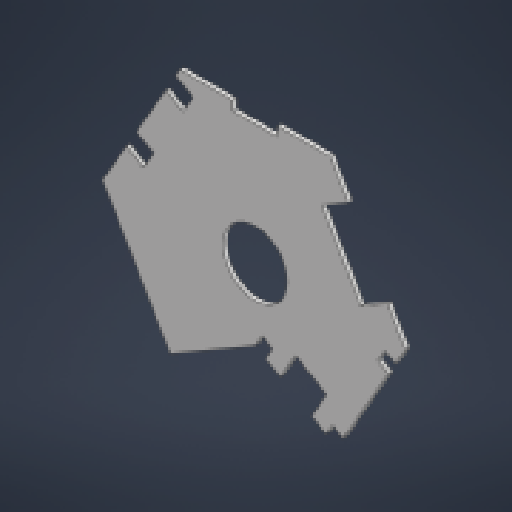
# Autodesk Inventor part: LilypadPCB
Saved by Autodesk Inventor 2023 (Build 270158000, 158)
## iProperties
Created: 2022-07-15
Part Number: LilypadPCB
Material: Generic
Document SubType Name: Modeling
Designer: jevan
Density: 1 g/cm^3
Appearance: Default
Author: jevan
Autodesk Inventor part; units mm, degrees
ref_plane "YZ Plane" through (0, 0, 0) normal (1, 0, 0) x (0, 1, 0)
ref_plane "XZ Plane" through (0, 0, 0) normal (0, 1, 0) x (-1, 0, 0)
ref_plane "XY Plane" through (0, 0, 0) normal (0, 0, 1) x (1, 0, 0)
sketch "Sketch1" plane through (0, 0, 0) normal (0, 0, 1) x (1, 0, 0)
  line L0 (37.2391, 0) -> (18.6195, -32.25)
  line L1 (18.6195, -32.25) -> (-18.6195, -32.25)
  line L2 (-18.6195, -32.25) -> (-37.2391, 0)
  line L3 (-37.2391, 0) -> (-18.6195, 32.25)
  line L4 (-18.6195, 32.25) -> (18.6195, 32.25)
  line L5 (18.6195, 32.25) -> (37.2391, 0)
  line L6 (18.6195, -32.25) -> (20.2545, -29.4181)
  line L7 (20.2545, -29.4181) -> (0, -17.7241)
  line L8 (0, -17.7241) -> (-20.2545, -29.4181)
  line L9 (-20.2545, -29.4181) -> (-21.1206, -29.9181)
  line L10 (-21.1206, -29.9181) -> (-37.8164, -1)
  line L11 (-37.8164, -1) -> (-37.2391, 0)
  circle A0 centre (0, 0) radius 8
  line L12 (-37.8164, -1) -> (-31.9414, 9.1758)
  line L13 (-31.9414, 9.1758) -> (-27.6806, 6.7158)
  line L14 (-27.6806, 6.7158) -> (-25.1806, 11.0459)
  line L15 (-25.1806, 11.0459) -> (-29.4414, 13.5059)
  line L16 (-29.4414, 13.5059) -> (-22.1914, 26.0633)
  line L17 (-22.1914, 26.0633) -> (-17.9133, 23.5933)
  line L18 (-17.9133, 23.5933) -> (-15.4133, 27.9234)
  line L19 (-15.4133, 27.9234) -> (-19.6914, 30.3934)
  line L20 (0, 32.25) -> (5.55, 32.25)
  line L21 (0, 32.25) -> (-5.55, 32.25)
  line L22 (-5.55, 32.25) -> (-5.55, 29.94)
  line L23 (-5.55, 29.94) -> (5.55, 29.94)
  line L24 (5.55, 29.94) -> (5.55, 32.25)
  line L25 (27.9293, 16.125) -> (32.7793, 7.7246)
  line L26 (27.9293, 16.125) -> (23.0793, 24.5254)
  line L27 (23.0793, 24.5254) -> (16.4975, 20.7254)
  line L28 (16.4975, 20.7254) -> (26.1975, 3.9246)
  line L29 (26.1975, 3.9246) -> (32.7793, 7.7246)
  line L30 (37.2391, 0) -> (34.7641, -4.2868)
  line L31 (34.7641, -4.2868) -> (32.1227, -2.7618)
  line L32 (32.1227, -2.7618) -> (30.4227, -5.7063)
  line L33 (30.4227, -5.7063) -> (33.0641, -7.2313)
  line L34 (33.0641, -7.2313) -> (21.8141, -26.7169)
  line L35 (21.8141, -26.7169) -> (19.1641, -25.1869)
  line L36 (19.1641, -25.1869) -> (17.6045, -27.8881)
  line L37 (10.1273, -23.5711) -> (13.9984, -25.8061)
  line L38 (10.1273, -23.5711) -> (6.2561, -21.3361)
  line L39 (6.2561, -21.3361) -> (9.9861, -14.8756)
  line L40 (9.9861, -14.8756) -> (17.7284, -19.3456)
  line L41 (17.7284, -19.3456) -> (13.9984, -25.8061)
  line L42 (6.2561, -21.3361) -> (2.6015, -19.2261)
  line L43 (2.6015, -19.2261) -> (4.3015, -16.2816)
  line L44 (4.3015, -16.2816) -> (1.7, -14.7796)
  line L45 (1.7, -14.7796) -> (0, -17.7241)
  dimension "d0" = 64.5
  dimension "d1" = 3.27
  dimension "d2" = 1
  dimension "d3" = 16
  dimension "d4" = 11.75
  dimension "d5" = 4.92
  dimension "d6" = 5
  dimension "d7" = 14.5
  dimension "d8" = 4.94
  dimension "d9" = 5
  dimension "d10" = 5.55
  dimension "d11" = 5.55
  dimension "d12" = 2.31
  dimension "d13" = 9.7
  dimension "d14" = 9.7
  dimension "d15" = 7.6
  dimension "d16" = 4.95
  dimension "d17" = 3.05
  dimension "d18" = 3.4
  dimension "d19" = 22.5
  dimension "d21" = 3.06
  dimension "d22" = 4.47
  dimension "d23" = 4.47
  dimension "d24" = 7.46
  dimension "d25" = 4.22
  dimension "d26" = 3.4
  constraints: 92 end point, 25 perpendicular, 19 point on line, 3 midpoint, 2 coincident, 2 parallel, 1 centre point, 1 equal length, 1 horizontal, 13 other
  measures "d0" distance between parallel lines of L3 L0
  measures "d1" distance of L0.end L6.end
  measures "d2" distance of L8.end L9.end
  measures "d3" diameter of A0
  measures "d4" distance of L10.end L12.end
  measures "d5" distance of L12.end L13.end
  measures "d6" distance of L13.end L14.end
  measures "d7" distance of L15.end L16.end
  measures "d8" distance of L16.end L17.end
  measures "d9" distance of L17.end L18.end
  measures "d10" distance of L20.start L20.end
  measures "d11" distance of L20.start L21.end
  measures "d12" distance of L21.end L22.end
  measures "d13" distance of L25.start L25.end
  measures "d14" distance of L25.start L26.end
  measures "d15" distance of L26.end L27.end
  measures "d16" distance of L0.start L30.end
  measures "d17" distance of L30.end L31.end
  measures "d18" distance of L31.end L32.end
  measures "d19" distance of L33.end L34.end
  measures "d21" distance of L34.end L35.end
  measures "d22" distance of L37.start L37.end
  measures "d23" distance of L37.start L38.end
  measures "d24" distance of L38.end L39.end
  measures "d25" distance of L38.end L42.end
  measures "d26" distance of L42.end L43.end
extrude "Extrusion1" add sketch "Sketch1" along normal blind 1 contours L0 L31 L32 L33 L35 L36 L7 L41 L40 L39 L43 L44 L45 L8 L2 L3 L13 L14 L15 L17 L18 L19 L4 L22 L23 L24 L5 L27 L28 L29 | L9 L10 L11 L2
body "Solid1"
